Autodesk Inventor part; units mm, degrees
(part 2 of 2)
sketch "Sketch31" plane through (0, 0, 0) normal (0, 0, -1) x (-1, 0, 0)
  circle A0 centre (14.15, -7.5) radius 1.5 projected
  line L0 (11.15, 4.6035) -> (11.15, 31) projected
  line L1 (11.15, 31) -> (44.35, 31) projected
  line L2 (44.35, 31) -> (44.35, 33) projected
  line L3 (44.35, 33) -> (103.65, 33) projected
  line L4 (103.65, 33) -> (103.65, -7) projected
  line L5 (103.65, -7) -> (44.35, -7) projected
  line L6 (44.35, -7) -> (44.35, -5) projected
  line L7 (44.35, -5) -> (11.15, -5) projected
  line L8 (11.15, -5) -> (11.15, -10.5) projected
  line L9 (11.15, -10.5) -> (19.9437, -10.5) projected
  arc A1 (11.15, 4.6035) -> (19.9437, -10.5) centre (0, -12) ccw projected
  circle A2 centre (14.15, 33.5) radius 1.5 projected
  circle A3 centre (107.15, -7.5) radius 1.5 projected
  circle A4 centre (107.15, 33.5) radius 1.5 projected
  circle A5 centre (58, -31) radius 1.5 projected
  circle A6 centre (28, -31) radius 1.5 projected
  circle A7 centre (-28, -31) radius 1.5 projected
  circle A8 centre (-58, -31) radius 1.5 projected
  line L10 (41.4971, -15.64) -> (41.4971, -12.79) projected
  line L11 (41.4971, -12.79) -> (49.9971, -12.79) projected
  line L12 (49.9971, -12.79) -> (49.9971, -14.59) projected
  line L13 (54.0971, -14.59) -> (54.0971, -12.79) projected
  line L14 (54.0971, -12.79) -> (62.5971, -12.79) projected
  line L15 (62.5971, -12.79) -> (62.5971, -15.64) projected
  line L16 (81.1492, -15.64) -> (81.1492, -12.19) projected
  line L17 (81.1492, -12.19) -> (93.3492, -12.19) projected
  line L18 (93.3492, -12.19) -> (93.3492, -15.64) projected
  line L19 (100.8492, -15.64) -> (100.8492, -18.89) projected
  line L20 (100.8492, -18.89) -> (33.4971, -18.89) projected
  line L21 (-97, -10) -> (-94.135, -10) projected
  line L22 (-94.135, -10) -> (-94.135, -8.15) projected
  line L23 (-94.135, -8.15) -> (-79.265, -8.15) projected
  line L24 (-79.265, -8.15) -> (-79.265, -10) projected
  line L25 (-79.265, -10) -> (-74.45, -10) projected
  line L26 (-74.45, -10) -> (-74.45, -7.4) projected
  line L27 (-74.45, -7.4) -> (-65.95, -7.4) projected
  line L28 (-65.95, -7.4) -> (-65.95, -10) projected
  line L29 (-65.95, -10) -> (-25, -10) projected
  line L30 (-25, -10) -> (-25, -11.5) projected
  line L31 (-25, -11.5) -> (-97, -11.5) projected
  line L32 (-97, -11.5) -> (-97, -10) projected
  line L33 (-24.3811, -2.4) -> (-40.7536, -2.4) projected
  arc A9 (-41.4091, 1.4895) -> (-40.7536, -2.4) centre (-40.7536, -0.4) ccw projected
  line L34 (-41.4091, 1.4895) -> (-19.7131, 9.0156) projected
  arc A10 (-17.6459, 5.7093) -> (-19.7131, 9.0156) centre (-19.0576, 7.1261) ccw projected
  arc A11 (-17.6459, 5.7093) -> (-22.5751, -1.2593) centre (0, -12) ccw projected
  arc A12 (-24.3811, -2.4) -> (-22.5751, -1.2593) centre (-24.3811, -0.4) ccw projected
  line L35 (-57.75, 3.9241) -> (-57.75, 16.5) projected
  arc A13 (-55.75, 18.5) -> (-57.75, 16.5) centre (-55.75, 16.5) ccw projected
  line L36 (-55.75, 18.5) -> (-19.4964, 18.5) projected
  arc A14 (-18.8409, 14.6105) -> (-19.4964, 18.5) centre (-19.4964, 16.5) ccw projected
  line L37 (-18.8409, 14.6105) -> (-55.0945, 2.0345) projected
  arc A15 (-57.75, 3.9241) -> (-55.0945, 2.0345) centre (-55.75, 3.9241) ccw projected
  arc A16 (-120.5, -0.4) -> (-118.5, -2.4) centre (-118.5, -0.4) ccw projected
  line L38 (-120.5, -0.4) -> (-120.5, 13.0432) projected
  arc A17 (-117.8445, 14.9327) -> (-120.5, 13.0432) centre (-118.5, 13.0432) ccw projected
  line L39 (-117.8445, 14.9327) -> (-79.0909, 1.4895) projected
  arc A18 (-79.7464, -2.4) -> (-79.0909, 1.4895) centre (-79.7464, -0.4) ccw projected
  line L40 (-79.7464, -2.4) -> (-118.5, -2.4) projected
  line L41 (-65.4055, 2.0345) -> (-101.6591, 14.6105) projected
  arc A19 (-101.0036, 18.5) -> (-101.6591, 14.6105) centre (-101.0036, 16.5) ccw projected
  line L42 (-101.0036, 18.5) -> (-64.75, 18.5) projected
  arc A20 (-62.75, 16.5) -> (-64.75, 18.5) centre (-64.75, 16.5) ccw projected
  line L43 (-62.75, 16.5) -> (-62.75, 3.9241) projected
  arc A21 (-65.4055, 2.0345) -> (-62.75, 3.9241) centre (-64.75, 3.9241) ccw projected
  line L44 (123, -7.178) -> (123, 29.5) projected
  line L45 (123, 29.5) -> (116.5, 29.5) projected
  line L46 (116.5, 29.5) -> (116.5, 36.5) projected
  line L47 (-45, 36.5) -> (116.5, 36.5) projected
  line L48 (-45, 36.5) -> (-45, 23.5) projected
  line L49 (-123, 23.5) -> (-45, 23.5) projected
  line L50 (-123, 23.5) -> (-123, -7.178) projected
  arc A22 (-123, -7.178) -> (-120.2885, -9.3426) centre (-115.5, -0.5637) ccw projected
  line L51 (-120.2885, -9.3426) -> (-69.9886, -36.779) projected
  arc A23 (-69.9886, -36.779) -> (-65.2001, -38) centre (-65.2001, -28) ccw projected
  line L52 (-65.2001, -38) -> (65.2001, -38) projected
  arc A24 (65.2001, -38) -> (69.9886, -36.779) centre (65.2001, -28) ccw projected
  line L53 (69.9886, -36.779) -> (120.2885, -9.3426) projected
  arc A25 (120.2885, -9.3426) -> (123, -7.178) centre (115.5, -0.5637) ccw projected
  line L54 (-25, -10) -> (-97, -10)
  line L55 (-97, -10) -> (-97, 0)
  line L56 (-97, 0) -> (-25, 0)
  line L57 (-25, 0) -> (-25, -10)
  line L58 (-97, -11.5) -> (-25, -11.5)
  line L59 (-25, -11.5) -> (-25, -14.5)
  line L60 (-25, -14.5) -> (-97, -14.5)
  line L61 (-97, -14.5) -> (-97, -11.5)
  line L62 (-82, -11.5) -> (-82, -14.5)
  line L63 (-35, -11.5) -> (-35, -14.5)
  line L64 (33.4971, -15.64) -> (41.4971, -15.64) projected
  line L65 (62.5971, -15.64) -> (81.1492, -15.64) projected
  line L66 (93.3492, -15.64) -> (100.8492, -15.64) projected
  line L67 (33.4971, -18.89) -> (33.4971, -15.64) projected
  line L68 (49.9971, -14.59) -> (54.0971, -14.59) projected
  point P0 (0, 0)
  point P1 (-25, -2.4)
  point P2 (-42.7132, 0)
  point P3 (-77.7868, 0)
  point P4 (-97, -2.4)
  point P5 (-82, -13)
  point P6 (-35, -11.5)
  dimension "d271" = 10
  dimension "d277" = 3
  dimension "d278" = 10
  dimension "d279" = 15
  constraints: 20 end point, 5 parallel, 4 point on line, 3 perpendicular, 2 horizontal, 2 vertical alignment, 1 midpoint
  measures "d271" distance between parallel lines of L54 L56
  measures "d277" distance of L58.end L59.end
  measures "d278" distance between parallel lines of L59 L63
  measures "d279" distance from line of point (-82, -13) L61
extrude "Extrusion28" cut sketch "Sketch31" against normal blind 4 contours L55 L40 A18 L56 A9 L33 L57 L29 L28 L27 L26 L25 L24 L23 L22 L21 | L31 L63 L60 L62
chamfer "Chamfer7" distance 9 distance2 4 1 edges at (60.25, 0, 0)
chamfer "Chamfer8" distance 3 angle 45 2 edges at (82, -14.5, 2) (35, -14.5, 2)
fillet "Fillet6" radius 3 2 edges at (97, -2.4, 2) (25, -2.4, 2)
chamfer "Chamfer9" distance 1.5 angle 45 6 edges at (-41.4971, -15.64, 2.5) (-62.5971, -15.64, 2.5) (-81.1492, -15.64, 2.5) (-93.3492, -15.64, 2.5) (-54.0971, -14.59, 2.5) (-49.9971, -14.59, 2.5)
chamfer "Chamfer10" distance 5 angle 45 2 edges at (-123, 14.661, 5) (123, 14.661, 5)
equation "\"d118\" = d117"
equation "\"d160\" = d158"
equation "\"d161\" = d159"
body "Solid1"
